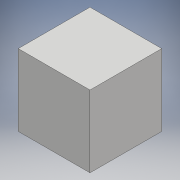
# Autodesk Inventor part: Cube
Saved by Autodesk Inventor 2018 (Build 220112000, 112)
## iProperties
Created: 2017-06-02
Part Number: Cube
Material: Generic
Document SubType Name: Modeling
Designer: Damian
Density: 1 g/cm^3
Appearance: Default
Author: Damian
Autodesk Inventor part; units mm, degrees
ref_plane "YZ Plane" through (0, 0, 0) normal (1, 0, 0) x (0, 1, 0)
ref_plane "XZ Plane" through (0, 0, 0) normal (0, 1, 0) x (-1, 0, 0)
ref_plane "XY Plane" through (0, 0, 0) normal (0, 0, 1) x (1, 0, 0)
sketch "Sketch1" plane through (0, 0, 0) normal (0, 1, 0) x (-1, 0, 0)
  line L0 (61.0294, 67.3203) -> (-88.9706, 67.3203)
  line L1 (-88.9706, 67.3203) -> (-88.9706, -82.6797)
  line L2 (-88.9706, -82.6797) -> (61.0294, -82.6797)
  line L3 (61.0294, -82.6797) -> (61.0294, 67.3203)
  point P0 (0, 0)
  dimension "d0" = 150
  constraints: 8 end point, 2 parallel, 2 perpendicular, 1 horizontal
  measures "d0" distance of L2.end L0.start
extrude "Extrusion1" add sketch "Sketch1" along normal blind 150
body "Solid1"
